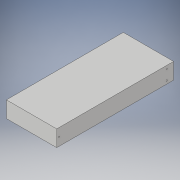
# Autodesk Inventor part: RSP-1000PS
Saved by Autodesk Inventor 2019 (Build 230136000, 136)
## iProperties
Created: 2019-05-23
Part Number: RSP-1000PS
Material: Generic
Document SubType Name: Modeling
Designer: Jorian Bruslind
Density: 1 g/cm^3
Appearance: Default
Author: Jorian Bruslind
Autodesk Inventor part; units mm, degrees
ref_plane "XZ Plane" through (0, 0, 0) normal (0, 1, 0) x (-1, 0, 0)
ref_plane "XY Plane" through (0, 0, 0) normal (0, 0, 1) x (1, 0, 0)
sketch "Sketch1" plane through (0, 0, 0) normal (0, 1, 0) x (-1, 0, 0)
  line L0 (0, 0) -> (127, 0)
  line L1 (127, 0) -> (127, -295)
  line L2 (127, -295) -> (0, -295)
  line L3 (0, -295) -> (0, 0)
  dimension "d0" = 127
  dimension "d1" = 295
  constraints: 8 end point, 2 parallel, 1 horizontal, 1 perpendicular
  measures "d0" distance of L1.end L2.end
  measures "d1" distance of L0.end L1.end
extrude "Extrusion1" add sketch "Sketch1" along normal blind 41
sketch "Sketch2" plane through (0, 0, 0) normal (1, 0, 0) x (0, 0, -1)
  line L0 (0, 0) -> (0, 20.5)
  line L1 (0, 0) -> (0, 41) projected
  line L2 (0, 20.5) -> (6, 20.5)
  circle A0 centre (6, 20.5) radius 1.75
  line L3 (295, 0) -> (0, 0) projected
  line L4 (295, 0) -> (295, 7.8)
  line L5 (295, 0) -> (295, 41) projected
  line L6 (0, 0) -> (277.7, 0)
  line L7 (277.7, 0) -> (277.7, 7.8)
  line L8 (277.7, 7.8) -> (277.7, 33.2)
  circle A1 centre (277.7, 7.8) radius 1.75
  circle A2 centre (277.7, 33.2) radius 1.75
  dimension "d4" = 20.5
  dimension "d5" = 6
  dimension "d6" = 3.5
  dimension "d7" = 7.8
  dimension "d8" = 277.7
  dimension "d9" = 7.8
  dimension "d10" = 25.4
  dimension "d11" = 3.5
  dimension "d12" = 3.5
  constraints: 12 end point, 3 centre point, 3 coincident, 3 point on line, 1 horizontal, 1 midpoint, 1 perpendicular
  measures "d4" distance of L0.start L0.end
  measures "d5" distance of L0.end L2.end
  measures "d6" diameter of A0
  measures "d7" distance of L3.start L4.end
  measures "d8" distance of L0.start L6.end
  measures "d9" distance of L6.end L7.end
  measures "d10" distance of L7.end L8.end
  measures "d11" diameter of A1
  measures "d12" diameter of A2
extrude "Extrusion2" cut sketch "Sketch2" against normal blind 10
ref_plane "Work Plane1" through (-63.5, 0, 0) normal (1, 0, 0) x (0, 1, 0)
mirror "Mirror1" about plane through (-63.5, 0, 0) normal (1, 0, 0) of "Extrusion2"
body "Solid1"
